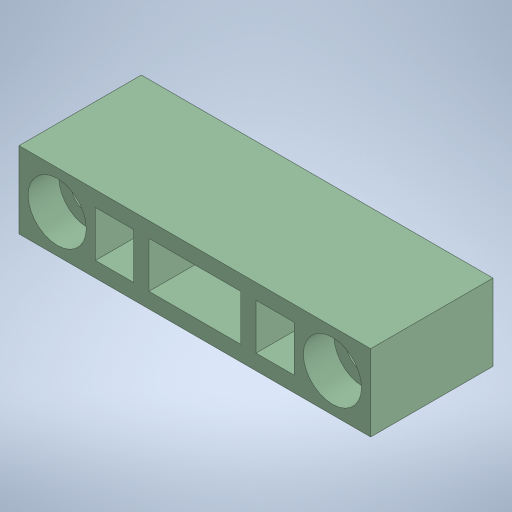
# Autodesk Inventor part: griper_TPU-2
Saved by Autodesk Inventor 2024 (Build 280153000, 153)
## iProperties
Created: 2025-06-05
Part Number: griper_TPU-2
Material: ゴム、シリコーン
Document SubType Name: Modeling
Designer: 1412z
Density: 1.25 g/cm^3
Appearance: ゴム - 緑
Author: 1412z
Autodesk Inventor part; units mm, degrees
ref_plane "YZ Plane" through (0, 0, 0) normal (1, 0, 0) x (0, 1, 0)
ref_plane "XZ Plane" through (0, 0, 0) normal (0, 1, 0) x (-1, 0, 0)
ref_plane "XY Plane" through (0, 0, 0) normal (0, 0, 1) x (1, 0, 0)
sketch "スケッチ1" plane through (0, 0, 0) normal (0, 0, 1) x (1, 0, 0)
  line L0 (-11.5, -2.5) -> (11.5, -2.5)
  line L1 (11.5, -2.5) -> (11.5, 2.5)
  line L2 (11.5, 2.5) -> (-11.5, 2.5)
  line L3 (-11.5, 2.5) -> (-11.5, -2.5)
  line L4 (-11.5, -2.5) -> (11.5, 2.5) construction
  line L5 (11.5, -2.5) -> (-11.5, 2.5) construction
  circle A0 centre (9, 0) radius 1.1
  circle A1 centre (-9, 0) radius 1.1
  line L6 (-11.5, -1.5) -> (11.5, -1.5)
  line L7 (11.5, 1.5) -> (-11.5, 1.5)
  line L8 (-6.5, -2.5) -> (-6.5, 2.5)
  line L9 (6.5, -2.5) -> (6.5, 2.5)
  line L10 (-4, -1.5) -> (-4, 1.5)
  line L11 (-3, -1.5) -> (-3, 1.5)
  line L12 (4, -1.5) -> (4, 1.5)
  line L13 (3, -1.5) -> (3, 1.5)
  point P0 (0, 0)
  point P1 (-6.5, -1.5)
  point P2 (-6.5, 1.5)
  point P3 (6.5, -1.5)
  point P4 (6.5, 1.5)
  dimension "d0" = 23
  dimension "d1" = 5
  dimension "d2" = 2.2
  dimension "d3" = 2.2
  dimension "d4" = 5
  dimension "d5" = 5
  constraints: 28 end point, 16 point on line, 9 perpendicular, 2 centre point, 2 midpoint, 2 parallel, 1 horizontal
  measures "d0" distance of L2.end L1.end
  measures "d1" distance of L1.end L0.end
  measures "d2" diameter of A0
  measures "d3" diameter of A1
  measures "d4" distance between parallel lines of L8 L3
  measures "d5" distance between parallel lines of L9 L1
extrude "押し出し1" add sketch "スケッチ1" along normal blind 8 contours L3 L6 L8 L0 | L8 L6 L9 L0 | L3 L7 L8 L6 | L9 L6 L1 L0 | L3 L2 L8 L7 | L9 L7 L1 L6 | L10 L7 L11 L6 | L8 L2 L9 L7 | L6 L13 L7 L12 | L9 L2 L1 L7
sketch "スケッチ2" plane through (0, 0, 8) normal (0, 0, 1) x (1, 0, 0)
  circle A0 centre (-9, 0) radius 1.1 projected
  circle A1 centre (-9, 0) radius 1.9
  circle A2 centre (9, 0) radius 1.1 projected
  circle A3 centre (9, 0) radius 1.9
  point P0 (0, 0)
  dimension "d8" = 3.8
  dimension "d9" = 3.8
  constraints: 2 centre point, 2 coincident
  measures "d8" diameter of A1
  measures "d9" diameter of A3
extrude "押し出し2" cut sketch "スケッチ2" against normal blind 2 contours A0 | A1 | A3
